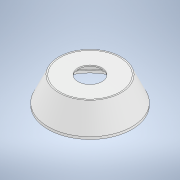
# Autodesk Inventor part: Parte baja R2D2
Saved by Autodesk Inventor 2022.2 (Build 262287010, 287A)
## iProperties
Created: 2022-10-09
Part Number: Parte baja R2D2
Material: Generic
Document SubType Name: Modeling
Designer: User
Density: 1 g/cm^3
Appearance: Default
Author: User
Autodesk Inventor part; units mm, degrees
ref_plane "YZ Plane" through (0, 0, 0) normal (1, 0, 0) x (0, 1, 0)
ref_plane "XZ Plane" through (0, 0, 0) normal (0, 1, 0) x (-1, 0, 0)
ref_plane "XY Plane" through (0, 0, 0) normal (0, 0, 1) x (1, 0, 0)
sketch "Sketch1" plane through (0, 0, 0) normal (0, 1, 0) x (-1, 0, 0)
  circle A0 centre (0, 0) radius 175
  circle A1 centre (0, 0) radius 165
  dimension "d0" = 350
  dimension "d1" = 10
  constraints: 2 centre point, 2 coincident
  measures "d0" diameter of A0
  measures "d1" radial gap between concentric circles of A0 A1
extrude "Extrusion1" add sketch "Sketch1" along normal blind 10
ref_plane "Work Plane1" through (0, 110, 0) normal (0, 1, 0) x (1, 0, 0)
sketch "Sketch2" plane through (0, 110, 0) normal (0, 1, 0) x (1, 0, 0)
  circle A0 centre (0, 0) radius 135
  circle A1 centre (0, 0) radius 165 projected
  circle A2 centre (0, 0) radius 130
  dimension "d5" = 30
  dimension "d6" = 5
  constraints: 2 centre point, 2 coincident
  measures "d5" radial gap between concentric circles of A0 A1
  measures "d6" radial gap between concentric circles of A0 A2
loft "Loft1" add profiles "Sketch2" section 1 edges at (175, 10, 0) contours A2
shell "Shell1" thickness 5 removed faces 2 at (13.8311, 110, -43.4771) at (57.1147, 10, 28.3555)
sketch "Sketch3" plane through (0, 110, 0) normal (0, 1, 0) x (1, 0, 0)
  circle A0 centre (0, 0) radius 50
  circle A1 centre (0, 0) radius 124.5171
  dimension "d14" = 100
  dimension "d15" = 74.5171
  constraints: 2 centre point, 2 coincident
  measures "d14" diameter of A0
  measures "d15" radial gap between concentric circles of A1 A0
extrude "Extrusion3" add sketch "Sketch3" against normal blind 5
body "Solid1"
